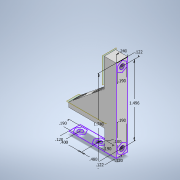
# Autodesk Inventor part: dispBracket
Saved by Autodesk Inventor 2020 (Build 240168000, 168)
## iProperties
Created: 2021-03-23
Part Number: dispBracket
Material: Generic
Document SubType Name: Modeling
Designer: rick
Density: 1 g/cm^3
Appearance: Default
Author: rick
Autodesk Inventor part; units mm, degrees
ref_plane "YZ Plane" through (0, 0, 0) normal (1, 0, 0) x (0, 1, 0)
ref_plane "XZ Plane" through (0, 0, 0) normal (0, 1, 0) x (-1, 0, 0)
ref_plane "XY Plane" through (0, 0, 0) normal (0, 0, 1) x (1, 0, 0)
sketch "Sketch1" plane through (0, 0, 0) normal (0, 0, 1) x (1, 0, 0)
  line L0 (0, 0) -> (-6.096, 0)
  line L1 (-6.096, 0) -> (-6.096, 10.922)
  line L2 (-6.096, 10.922) -> (-25.4, 10.922)
  line L3 (-25.4, 10.922) -> (-25.4, 13.462)
  line L4 (-25.4, 13.462) -> (-6.35, 28.956)
  line L5 (-6.35, 28.956) -> (-6.35, 44.196)
  line L6 (-6.35, 44.196) -> (0, 44.196)
  line L7 (0, 44.196) -> (0, 0)
  dimension "d0" = 44.196
  dimension "d1" = 10.922
  dimension "d2" = 2.54
  dimension "d3" = 19.304
  dimension "d4" = 15.24
  dimension "d25" = 6.35
  constraints: 16 end point, 5 perpendicular, 1 horizontal, 1 parallel
  measures "d0" distance of L6.end L0.start
  measures "d1" distance of L0.end L1.end
  measures "d2" distance of L2.end L3.end
  measures "d3" distance of L1.end L2.end
  measures "d4" distance of L4.end L5.end
  measures "d25" distance of L5.end L6.end
sketch "Sketch2" plane through (0, 0, 0) normal (1, 0, 0) x (0, 1, 0)
  line L0 (0, 3.048) -> (0, -3.048)
  line L1 (0, -3.048) -> (44.196, -3.048)
  line L2 (44.196, -3.048) -> (44.196, 3.048)
  line L3 (44.196, 3.048) -> (0, 3.048)
  circle A0 centre (3.0988, 0) radius 1.2762
  circle A1 centre (41.0972, 0) radius 1.2712
  line L4 (38.3109, 0) -> (39.7041, 2.413)
  line L5 (39.7041, 2.413) -> (42.4903, 2.413)
  line L6 (42.4903, 2.413) -> (43.8835, 0)
  line L7 (43.8835, 0) -> (42.4903, -2.413)
  line L8 (42.4903, -2.413) -> (39.7041, -2.413)
  line L9 (39.7041, -2.413) -> (38.3109, 0)
  line L10 (5.8851, -0.001) -> (4.4911, -2.4135)
  line L11 (4.4911, -2.4135) -> (1.7048, -2.4125)
  line L12 (1.7048, -2.4125) -> (0.3125, 0.001)
  line L13 (0.3125, 0.001) -> (1.7065, 2.4135)
  line L14 (1.7065, 2.4135) -> (4.4928, 2.4125)
  line L15 (4.4928, 2.4125) -> (5.8851, -0.001)
  point P0 (0, 0)
  dimension "d6" = 37.9984
  dimension "d7" = 3.0988
  dimension "d8" = 3.0988
  dimension "d9" = 44.196
  dimension "d10" = 4.826
  dimension "d11" = 6.096
  dimension "d12" = 3.048
  dimension "d13" = 4.826
  constraints: 32 end point, 3 perpendicular, 2 centre point, 2 coincident, 1 vertical, 2 other
  measures "d6" distance of A1.centre A0.centre
  measures "d7" distance from line of L2 A1.centre
  measures "d8" distance from line of L0 A0.centre
  measures "d9" distance from line of point (0, 0) L2
  measures "d10" distance between parallel lines of L5 L8
  measures "d11" distance of L1.end L2.end
  measures "d12" distance of L0.start point (0, 0)
  measures "d13" distance between parallel lines of L14 L11
sketch "Sketch3" plane through (0, 0, 0) normal (0, 1, 0) x (-1, 0, 0)
  line L0 (0, -3.048) -> (0, 3.048)
  line L1 (0, 3.048) -> (25.4, 3.048)
  line L2 (25.4, 3.048) -> (25.4, -3.048)
  line L3 (25.4, -3.048) -> (0, -3.048)
  circle A0 centre (22.352, 0) radius 1.27
  circle A1 centre (12.192, 0) radius 1.27
  line L4 (19.5657, 0) -> (20.9589, 2.413)
  line L5 (20.9589, 2.413) -> (23.7451, 2.413)
  line L6 (23.7451, 2.413) -> (25.1383, 0)
  line L7 (25.1383, 0) -> (23.7451, -2.413)
  line L8 (23.7451, -2.413) -> (20.9589, -2.413)
  line L9 (20.9589, -2.413) -> (19.5657, 0)
  line L10 (9.4057, 0) -> (10.7989, 2.413)
  line L11 (10.7989, 2.413) -> (13.5851, 2.413)
  line L12 (13.5851, 2.413) -> (14.9783, 0)
  line L13 (14.9783, 0) -> (13.5851, -2.413)
  line L14 (13.5851, -2.413) -> (10.7989, -2.413)
  line L15 (10.7989, -2.413) -> (9.4057, 0)
  point P0 (0, 0)
  dimension "d14" = 12.192
  dimension "d15" = 10.16
  dimension "d16" = 3.048
  dimension "d17" = 2.54
  dimension "d18" = 4.826
  dimension "d19" = 4.826
  constraints: 32 end point, 2 centre point, 2 coincident, 2 perpendicular, 1 horizontal, 1 vertical, 26 other
  measures "d14" distance of point (0, 0) A1.centre
  measures "d15" distance of A0.centre A1.centre
  measures "d16" distance from line of L2 A0.centre
  measures "d17" diameter of A1
  measures "d18" distance between parallel lines of L5 L8
  measures "d19" distance between parallel lines of L11 L14
extrude "Extrusion1" add sketch "Sketch1" along normal mid plane 6.096
ref_plane "Work Plane1" through (-6.35, 28.956, 3.048) normal (-1, 0, 0) x (0, 0, 1)
extrude "Extrusion2" cut sketch "Sketch2" along normal blind 3.81 from surface at -6.35 contours A1 | L4 L5 L6 L7 L8 L9
extrude "Extrusion3" cut sketch "Sketch2" along normal blind 3.81 from surface at -6.35 contours A0 | L10 L11 L12 L13 L14 L15
hole "Hole1" at (0, 3.0988, 0) at (0, 41.0972, 0) direction (-1, 0, 0) diameter 2.54 end through all
ref_plane "Work Plane2" through (-25.4, 13.462, -3.048) normal (0, -1, 0) x (1, 0, 0)
extrude "Extrusion4" cut sketch "Sketch3" along normal blind 15.24 from surface at 13.462 contours A0 | A1 | L4 L5 L6 L7 L8 L9 | L10 L11 L12 L13 L14 L15
hole "Hole2" at (-22.352, 0, 0) at (-12.192, 0, 0) direction (0, 1, 0) diameter 2.54 end through all
body "Solid1"
